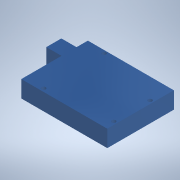
# Autodesk Inventor part: Arduino
Saved by Autodesk Inventor 2020 (Build 240168000, 168)
## iProperties
Created: 2020-01-26
Part Number: Arduino
Material: Generic
Document SubType Name: Modeling
Designer: holtat
Density: 1 g/cm^3
Appearance: Flaked Satin - Blue
Author: holtat
Autodesk Inventor part; units mm, degrees
ref_plane "YZ Plane" through (0, 0, 0) normal (1, 0, 0) x (0, 1, 0)
ref_plane "XZ Plane" through (0, 0, 0) normal (0, 1, 0) x (-1, 0, 0)
ref_plane "XY Plane" through (0, 0, 0) normal (0, 0, 1) x (1, 0, 0)
sketch "Sketch1" plane through (0, 0, 0) normal (0, 1, 0) x (-1, 0, 0)
  line L0 (34.29, -26.543) -> (-34.29, -26.543)
  line L1 (-34.29, -26.543) -> (-34.29, 26.543)
  line L2 (-34.29, 26.543) -> (34.29, 26.543)
  line L3 (34.29, 26.543) -> (34.29, -26.543)
  line L4 (34.29, -17.5006) -> (46.3824, -17.5006)
  line L5 (46.3824, -17.5006) -> (46.3824, -5.5118)
  line L6 (46.3824, -5.5118) -> (34.29, -5.5118)
  line L7 (34.29, -5.5118) -> (34.29, -17.5006)
  point P0 (0, 0)
  point P1 (0, -26.543)
  point P2 (34.29, 0)
  dimension "d0" = 68.58
  dimension "d1" = 53.086
  dimension "d2" = 9.0424
  dimension "d3" = 11.9888
  constraints: 16 end point, 4 parallel, 2 horizontal, 2 midpoint, 2 perpendicular, 1 horizontal alignment, 1 point on line, 1 vertical alignment
  measures "d0" distance of L0.start L0.end
  measures "d1" distance of L2.end L0.start
  measures "d2" distance between parallel lines of L0 L4
  measures "d3" distance of L4.end L5.end
extrude "Extrusion1" add sketch "Sketch1" along normal blind 13.3858
sketch "Sketch2" plane through (0, 13.3858, 0) normal (0, 1, 0) x (1, 0, 0)
  circle A0 centre (-19.05, 24.2401) radius 1.5875
  circle A1 centre (31.75, 10.033) radius 1.5875
  circle A2 centre (31.75, -18.923) radius 1.5875
  circle A3 centre (-19.05, -24.003) radius 1.5875
  line L0 (-34.29, 26.543) -> (-34.29, 17.5006) projected
  line L1 (34.29, -26.543) -> (34.29, 26.543) projected
  line L2 (34.29, 26.543) -> (-34.29, 26.543) projected
  line L3 (-34.29, -26.543) -> (34.29, -26.543) projected
  point P0 (0, 0)
  dimension "d6" = 15.24
  dimension "d7" = 3.175
  dimension "d9" = 16.51
  dimension "d10" = 7.62
  dimension "d11" = 2.54
  dimension "d12" = 50.8
  constraints: 4 centre point, 3 equal radius, 2 vertical alignment
  measures "d6" distance from line of L0 A0.centre
  measures "d7" diameter of A0
  measures "d9" distance from line of L2 A1.centre
  measures "d10" distance from line of L3 A2.centre
  measures "d11" distance from line of L3 A3.centre
  measures "d12" horizontal distance of A1.centre A0.centre
extrude "Extrusion2" cut sketch "Sketch2" against normal blind 13.3858
body "Solid1"
